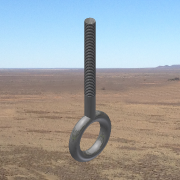
# Autodesk Inventor part: 0eye_ss_375
Saved by Autodesk Inventor 2013 SP2 (Build 170200200, 200)
## iProperties
Company: HERA Project
Created: 2013-07-11
Part Number: 0eye_ss_375
Material: Stainless Steel
Document SubType Name: Modeling
Designer: Dave
Mass: 125.152 g
Surface Area: 65.1863 cm^2
Volume: 15.4891 cm^3
Density: 8.08 g/cm^3
Description: 0.375 stainless eyebolt
Author: David DeBoer
Autodesk Inventor part; units mm, degrees
ref_plane "YZ Plane" through (0, 0, 0) normal (1, 0, 0) x (0, 1, 0)
ref_plane "XZ Plane" through (0, 0, 0) normal (0, 1, 0) x (-1, 0, 0)
sketch "Sketch1" plane through (0, 0, 0) normal (0, 1, 0) x (-1, 0, 0)
  circle A0 centre (0, 0) radius 4.7625
  dimension "d0" = 9.525
  constraints: 1 centre point, 1 coincident
  measures "d0" diameter of A0
extrude "Extrusion1" add sketch "Sketch1" along normal blind 101.6
thread "Thread4" size "3/8-16 UNC" class "2A" standard "ANSI Unified Screw Threads" length 76.2
sketch "Sketch2" plane through (0, 0, 0) normal (0, -1, 0) x (1, 0, 0)
  circle A0 centre (0, 0) radius 4.7625 projected
  point P0 (0, 4.7625)
  constraints: 1 vertical alignment, 1 other
ref_plane "Work Plane1" through (0, 0, 4.7625) normal (0, 0, 1) x (1, 0, 0)
ref_plane "Work Plane2" through (0, 0, 0) normal (0, 0, 1) x (1, 0, 0)
sketch "Sketch5" plane through (0, 0, 0) normal (0, 0, 1) x (1, 0, 0)
  circle A0 centre (0, 0) radius 4.7625
  line L0 (-4.7625, -19.05) -> (4.7625, -19.05)
  line L1 (-4.7625, 0) -> (4.7625, 0) projected
  dimension "d17" = 9.525
  dimension "d18" = 19.05
  constraints: 2 end point, 1 centre point, 1 coincident, 1 horizontal
  measures "d17" distance of L0.start L0.end
  measures "d18" distance between parallel lines of L0 L1
revolve "Revolution1" add sketch "Sketch5" angle 360 about axis through (-4.7625, -19.05, 0) along (1, 0, 0)
body "Solid1"
